Autodesk Inventor part; units mm, degrees
(part 3 of 3)
  line L1079 (126.5366, 52.0058) -> (124.6494, 53.4849) construction
  line L1080 (124.6494, 53.4849) -> (122.5377, 54.7805) construction
  line L1081 (122.5377, 54.7805) -> (120.9565, 55.6272) construction
  line L1082 (120.9565, 55.6272) -> (119.3753, 56.1475) construction
  line L1083 (119.3753, 56.1475) -> (116.8454, 56.3719) construction
  line L1084 (116.8454, 56.3719) -> (115.9477, 56.4535) construction
  line L1085 (115.9477, 56.4535) -> (115.7296, 56.3364) construction
  spline S44 degree 4 poles (121.3764, 52.0329) (122.5555, 51.423) (124.3304, 50.7304) (126.2568, 50.2109) (128.0317, 49.7347) (128.1688, 49.8533) (128.3423, 50.0879) (127.9036, 50.6184) (126.5366, 52.0058) (124.6494, 53.4849) (122.5377, 54.7805) (120.9565, 55.6272) (119.3753, 56.1475) (116.8454, 56.3719) (115.9477, 56.4535) (115.7296, 56.3364) knots 1 1 1 1 1 2 3 4 5 6 7 8 9 10 11 12 13 13 13 13 13
  line L1086 (112.9548, 57.8411) -> (112.0262, 58.7513) construction
  line L1087 (112.0262, 58.7513) -> (109.7638, 60.8045) construction
  line L1088 (109.7638, 60.8045) -> (107.9587, 62.1806) construction
  line L1089 (107.9587, 62.1806) -> (106.3363, 63.2029) construction
  line L1090 (106.3363, 63.2029) -> (104.7139, 64.492) construction
  line L1091 (104.7139, 64.492) -> (103.2248, 65.2699) construction
  line L1092 (103.2248, 65.2699) -> (102.6914, 65.4699) construction
  line L1093 (102.6914, 65.4699) -> (101.9802, 65.2254) construction
  line L1094 (101.9802, 65.2254) -> (101.4246, 64.9365) construction
  line L1095 (101.4246, 64.9365) -> (101.1135, 64.4698) construction
  line L1096 (101.1135, 64.4698) -> (101.069, 63.114) construction
  line L1097 (101.069, 63.114) -> (100.9579, 62.1584) construction
  line L1098 (100.9579, 62.1584) -> (100.9801, 61.425) construction
  line L1099 (100.9801, 61.425) -> (101.2246, 60.6249) construction
  line L1100 (101.2246, 60.6249) -> (101.1374, 60.3751) construction
  spline S45 degree 4 poles (112.9548, 57.8411) (112.0262, 58.7513) (109.7638, 60.8045) (107.9587, 62.1806) (106.3363, 63.2029) (104.7139, 64.492) (103.2248, 65.2699) (102.6914, 65.4699) (101.9802, 65.2254) (101.4246, 64.9365) (101.1135, 64.4698) (101.069, 63.114) (100.9579, 62.1584) (100.9801, 61.425) (101.2246, 60.6249) (101.1374, 60.3751) knots 1 1 1 1 1 2 3 4 5 6 7 8 9 10 11 12 13 13 13 13 13
  point P0 (0, 0)
  point P1 (50.6587, 35.9945)
  point P2 (113.2132, 42.5719)
  dimension "d72" = 3.302
  dimension "d66" = 3.302
  dimension "d67" = 3.302
  dimension "d68" = 3.302
  dimension "d69" = 3.302
  dimension "d70" = 3.302
  dimension "d71" = 3.302
  dimension "d73" = 3.302
  dimension "d74" = 3.302
  dimension "d75" = 3.302
  dimension "d76" = 3.302
  dimension "d77" = 3.302
  dimension "d78" = 3.302
  dimension "d79" = 3.302
  dimension "d80" = 3.302
  dimension "d81" = 3.302
  dimension "d82" = 3.302
  dimension "d83" = 3.302
  dimension "d84" = 3.302
  dimension "d85" = 3.302
  dimension "d86" = 3.302
  dimension "d87" = 3.302
  dimension "d88" = 3.302
  dimension "d89" = 3.302
  dimension "d90" = 3.302
  dimension "d91" = 3.302
  dimension "d92" = 3.302
  dimension "d93" = 3.302
  dimension "d94" = 3.302
  dimension "d95" = 3.302
  dimension "d96" = 3.302
  dimension "d97" = 3.302
  dimension "d98" = 3.302
  dimension "d99" = 3.302
  dimension "d100" = 3.302
  dimension "d101" = 3.302
  dimension "d102" = 0.762
  dimension "d103" = 0.762
  dimension "d105" = 0.762
  dimension "d107" = 0.762
  dimension "d108" = 0.762
  dimension "d109" = 0.762
  dimension "d110" = 0.762
  dimension "d111" = 0.762
  dimension "d112" = 0.762
  dimension "d113" = 0.762
  dimension "d114" = 0.762
  dimension "d115" = 0.762
  dimension "d116" = 0.762
  dimension "d117" = 0.762
  dimension "d119" = 0.762
  dimension "d120" = 0.762
  dimension "d121" = 0.762
  dimension "d122" = 0.762
  dimension "d123" = 0.762
  dimension "d124" = 0.762
  dimension "d125" = 0.762
  dimension "d126" = 0.762
  dimension "d127" = 0.762
  dimension "d128" = 0.762
  dimension "d129" = 0.762
  dimension "d131" = 0.762
  dimension "d132" = 0.762
  dimension "d133" = 0.762
  dimension "d135" = 0.762
  constraints: 94 point on circle, 71 centre point, 52 horizontal, 25 vertical, 3 tangent, 2 end point, 133 other
  measures "d66" diameter of A0
  measures "d67" diameter of A1
  measures "d68" diameter of A2
  measures "d69" diameter of A3
  measures "d70" diameter of A4
  measures "d71" diameter of A5
  measures "d73" diameter of A7
  measures "d74" diameter of A8
  measures "d75" diameter of A9
  measures "d76" diameter of A10
  measures "d77" diameter of A11
  measures "d78" diameter of A12
  measures "d79" diameter of A13
  measures "d80" diameter of A14
  measures "d81" diameter of A15
  measures "d82" diameter of A16
  measures "d83" diameter of A17
  measures "d84" diameter of A18
  measures "d85" diameter of A19
  measures "d86" diameter of A20
  measures "d87" diameter of A21
  measures "d88" diameter of A22
  measures "d89" diameter of A23
  measures "d90" diameter of A24
  measures "d91" diameter of A25
  measures "d92" diameter of A26
  measures "d93" diameter of A27
  measures "d94" diameter of A28
  measures "d95" diameter of A29
  measures "d96" diameter of A30
  measures "d97" diameter of A31
  measures "d98" diameter of A32
  measures "d99" diameter of A33
  measures "d100" diameter of A34
  measures "d101" diameter of A35
  measures "d102" radial gap between concentric circles of A0 A36
  measures "d103" radial gap between concentric circles of A2 A37
  measures "d105" radial gap between concentric circles of A4 A38
  measures "d107" radial gap between concentric circles of A5 A39
  measures "d109" radial gap between concentric circles of A15 A41
  measures "d110" radial gap between concentric circles of A16 A42
  measures "d111" radial gap between concentric circles of A17 A43
  measures "d112" radial gap between concentric circles of A19 A44
  measures "d113" radial gap between concentric circles of A18 A45
  measures "d114" radial gap between concentric circles of A22 A46
  measures "d115" radial gap between concentric circles of A7 A47
  measures "d116" radial gap between concentric circles of A1 A48
  measures "d117" radial gap between concentric circles of A3 A49
  measures "d119" radial gap between concentric circles of A24 A50
  measures "d120" radial gap between concentric circles of A23 A51
  measures "d121" radial gap between concentric circles of A20 A52
  measures "d122" radial gap between concentric circles of A21 A53
  measures "d123" radial gap between concentric circles of A28 A54
  measures "d124" radial gap between concentric circles of A27 A55
  measures "d125" radial gap between concentric circles of A29 A56
  measures "d126" radial gap between concentric circles of A30 A57
  measures "d127" radial gap between concentric circles of A26 A58
  measures "d128" radial gap between concentric circles of A25 A59
  measures "d129" radial gap between concentric circles of A9 A60
  measures "d131" radial gap between concentric circles of A10 A61
  measures "d132" radial gap between concentric circles of A11 A62
  measures "d133" radial gap between concentric circles of A13 A63
  measures "d135" radial gap between concentric circles of A14 A64
body "Solid2"
